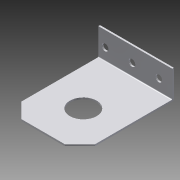
# Autodesk Inventor part: alignmentWheelsBarP2
Saved by Autodesk Inventor 2015 (Build 190159000, 159)
## iProperties
Created: 2015-01-30
Part Number: alignmentWheelsBarP2
Material: Generic
Document SubType Name: Modeling
Designer: Kingbob26
Density: 1 g/cm^3
Appearance: Default
Author: Kingbob26
Autodesk Inventor part; units mm, degrees
ref_plane "YZ Plane" through (0, 0, 0) normal (1, 0, 0) x (0, 1, 0)
ref_plane "XZ Plane" through (0, 0, 0) normal (0, 1, 0) x (-1, 0, 0)
ref_plane "XY Plane" through (0, 0, 0) normal (0, 0, 1) x (1, 0, 0)
sketch "Sketch1" plane through (0, 0, 0) normal (0, 1, 0) x (-1, 0, 0)
  line L0 (69.85, 88.9) -> (0, 88.9)
  line L1 (0, 88.9) -> (0, 0)
  line L2 (0, 0) -> (69.85, 0)
  line L3 (69.85, 0) -> (69.85, 88.9)
  constraints: 8 end point, 2 parallel, 1 horizontal, 1 perpendicular
extrude "Extrusion1" add sketch "Sketch1" along normal blind 1.5875
chamfer "Chamfer1" distance 14.2875 angle 45 1 edges at (-69.85, 0.7937, 88.9)
chamfer "Chamfer2" distance 14.2875 angle 45 1 edges at (0, 0.7937, 88.9)
sketch "Sketch2" plane through (0, 0, 0) normal (0, 0, -1) x (-1, 0, 0)
  line L0 (69.85, 26.9875) -> (0, 26.9875)
  line L1 (0, 26.9875) -> (0, 0)
  line L2 (0, 0) -> (69.85, 0)
  line L3 (69.85, 0) -> (69.85, 26.9875)
  constraints: 8 end point, 2 parallel, 1 horizontal, 1 perpendicular
sketch "Sketch3" plane through (0, 0, 0) normal (1, 0, 0) x (0, 0, -1)
  line L0 (0, 0) -> (-1.5875, 0)
  line L1 (-1.5875, 0) -> (-1.5875, 1.5875)
  line L2 (-1.5875, 1.5875) -> (0, 1.5875)
  line L3 (0, 1.5875) -> (0, 0)
  dimension "d8" = 1.5875
  dimension "d9" = 1.5875
  constraints: 8 end point, 2 parallel, 1 horizontal, 1 perpendicular
  measures "d8" distance of L1.end L2.end
  measures "d9" distance of L0.end L1.end
extrude "Extrusion2" cut sketch "Sketch3" against normal blind 69.85
extrude "Extrusion3" add sketch "Sketch2" against normal blind 1.5875
fillet "Fillet1" radius 0.7937 1 edges at (-34.925, 1.5875, 1.5875)
fillet "Fillet2" radius 0.7937 1 edges at (-34.925, 0, 0)
sketch "Sketch4" plane through (0, 0, 0) normal (0, 0, -1) x (-1, 0, 0)
  circle A0 centre (12.7, 12.7) radius 3.175
  point P0 (0, 0)
  dimension "d16" = 6.35
  constraints: 1 centre point
  measures "d16" diameter of A0
extrude "Extrusion4" cut sketch "Sketch4" against normal blind 1.5875
sketch "Sketch5" plane through (0, 0, 0) normal (0, 0, -1) x (-1, 0, 0)
  circle A0 centre (63.5, 12.7) radius 3.175
  point P0 (0, 0)
  dimension "d19" = 6.35
  constraints: 1 centre point
  measures "d19" diameter of A0
extrude "Extrusion5" cut sketch "Sketch5" against normal blind 1.5875
sketch "Sketch6" plane through (0, 0, 0) normal (0, 0, -1) x (-1, 0, 0)
  circle A0 centre (38.1, 12.7) radius 3.175
  point P0 (0, 0)
  dimension "d22" = 6.35
  constraints: 1 centre point
  measures "d22" diameter of A0
extrude "Extrusion6" cut sketch "Sketch6" against normal blind 1.5875
sketch "Sketch7" plane through (0, 0, 0) normal (0, -1, 0) x (1, 0, 0)
  circle A0 centre (-34.925, 50.8) radius 12.7
  point P0 (0, 0)
  dimension "d25" = 25.4
  constraints: 1 centre point
  measures "d25" diameter of A0
extrude "Extrusion7" cut sketch "Sketch7" against normal blind 1.5875
body "Solid1"
